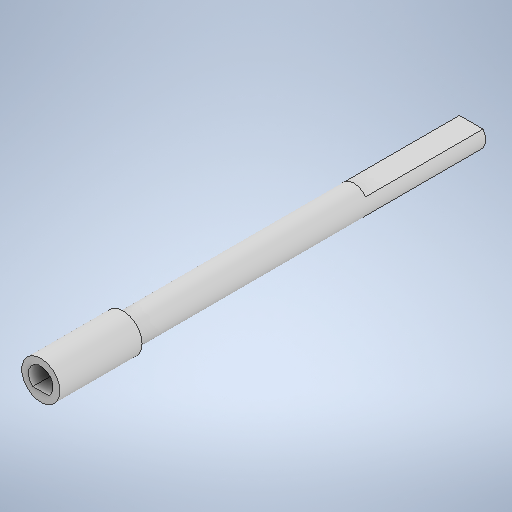
# Autodesk Inventor part: 13042026-08
Saved by Autodesk Inventor 2025.2 (Build 292293000, 293)
## iProperties
Created: 2026-05-06
Part Number: 13042026-08
Material: Generic
Document SubType Name: Modeling
Designer: Oski
Density: 1 g/cm^3
Appearance: Default
Author: Oski
Autodesk Inventor part; units mm, degrees
ref_plane "YZ Plane" through (0, 0, 0) normal (1, 0, 0) x (0, 1, 0)
ref_plane "XZ Plane" through (0, 0, 0) normal (0, 1, 0) x (-1, 0, 0)
ref_plane "XY Plane" through (0, 0, 0) normal (0, 0, 1) x (1, 0, 0)
sketch "Sketch1" plane through (0, 0, 0) normal (0, 0, 1) x (1, 0, 0)
  circle A0 centre (0, 0) radius 3.25
  dimension "d0" = 6.5
  constraints: 1 centre point, 1 coincident
  measures "d0" diameter of A0
extrude "Extrusion1" add sketch "Sketch1" along normal mid plane 14
sketch "Sketch2" plane through (0, 0, 7) normal (0, 0, 1) x (1, 0, 0)
  arc A0 (1.3601, -1.6) -> (-1.3601, -1.6) centre (0, 0) ccw
  line L0 (-1.3601, -1.6) -> (1.3601, -1.6)
  point P0 (0, 2.2)
  point P1 (0, -1.65)
  point P2 (0, -1.6)
  point P3 (0, 2.1)
  dimension "d4" = 2.1
  dimension "d12" = 3.7
  constraints: 3 point on circle, 2 end point, 1 centre point, 1 coincident, 1 horizontal, 1 midpoint
  measures "d4" radius of A0
  measures "d12" distance of point (0, -1.6) point (0, 2.1)
extrude "Extrusion2" cut sketch "Sketch2" against normal blind 8.5
sketch "Sketch3" plane through (0, 0, -7) normal (0, 0, -1) x (-1, 0, 0)
  circle A0 centre (0, 0) radius 2.45
  dimension "d9" = 4.9
  constraints: 1 centre point, 1 coincident
  measures "d9" diameter of A0
extrude "Extrusion3" add sketch "Sketch3" along normal blind 39.3
sketch "Sketch4" plane through (0, 0, -46.3) normal (0, 0, -1) x (-1, 0, 0)
  circle A0 centre (0, 0) radius 2.45 projected
  arc A1 (-2.0106, 1.4) -> (-2.0106, -1.4) centre (0, 0) ccw
  arc A2 (2.0106, -1.4) -> (2.0106, 1.4) centre (0, 0) ccw
  line L0 (-2.0106, 1.4) -> (2.0106, 1.4)
  line L1 (2.0106, -1.4) -> (-2.0106, -1.4)
  dimension "d13" = 1.4
  constraints: 8 point on circle, 4 end point, 2 centre point, 2 coincident, 2 parallel, 1 horizontal
  measures "d13" distance from line of L0 point (0, 0)
extrude "Extrusion4" add sketch "Sketch4" along normal blind 20 contours A0 L1 L0
body "Solid1"
